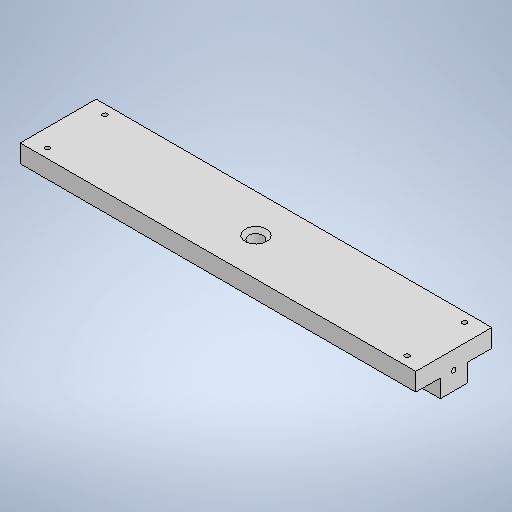
# Autodesk Inventor part: caster_holder
Saved by Autodesk Inventor 2026.3 (Build 303398000, 398)
## iProperties
Created: 2026-06-06
Part Number: caster_holder
Material: Generic
Document SubType Name: Modeling
Designer: gakut
Density: 1 g/cm^3
Appearance: Default
Author: gakut
## iProperties of the stored document caster_holder_3DPrint.ipt
Created: 2026-06-06
Part Number: caster_holder_3DPrint
Material: Generic
Document SubType Name: Modeling
Designer: gakut
Density: 1 g/cm^3
Appearance: Default
Author: gakut
Autodesk Inventor part; units mm, degrees
ref_plane "YZ Plane" through (0, 0, 0) normal (1, 0, 0) x (0, 1, 0)
ref_plane "XZ Plane" through (0, 0, 0) normal (0, 1, 0) x (-1, 0, 0)
ref_plane "XY Plane" through (0, 0, 0) normal (0, 0, 1) x (1, 0, 0)
sketch "Sketch1" plane through (0, 0, 0) normal (0, 1, 0) x (-1, 0, 0)
  line L0 (110, 21.125) -> (-110, 21.125)
  line L1 (-110, 21.125) -> (-110, -21.125)
  line L2 (-110, -21.125) -> (110, -21.125)
  line L3 (110, -21.125) -> (110, 21.125)
  line L4 (110, 21.125) -> (-110, -21.125) construction
  line L5 (-110, 21.125) -> (110, -21.125) construction
  point P0 (0, 0)
  dimension "d0" = 42.25
  dimension "d1" = 220
  constraints: 12 end point, 2 midpoint, 2 parallel, 1 horizontal, 1 perpendicular
  measures "d0" distance of L0.end L1.end
  measures "d1" distance of L0.start L0.end
extrude "Extrusion1" add sketch "Sketch1" along normal mid plane 20
sketch "Sketch2" plane through (0, 10, 0) normal (0, 1, 0) x (1, 0, 0)
  line L0 (110, 21.125) -> (-110, 21.125) projected
  line L1 (-110, -21.125) -> (110, -21.125) projected
  line L2 (-110, 21.125) -> (-110, -21.125) projected
  point P0 (0, 0)
  point P1 (-100, -16)
  point P2 (-100, 16)
  point P3 (-110, 0)
  dimension "d4" = 10
  dimension "d5" = 32
  dimension "d6" = 16
  constraints: 1 midpoint, 1 vertical alignment
  measures "d4" distance from line of L2 point (-100, 16)
  measures "d5" distance of point (-100, -16) point (-100, 16)
  measures "d6" vertical distance of point (-110, 0) point (-100, 16)
hole "Hole1" at (-100, 10, 16) at (-100, 10, -16) direction (0, -1, 0) diameter 2.6 end through all
mirror "Mirror1" about plane through (0, 0, 0) normal (1, 0, 0) of "Hole1"
sketch "Sketch4" plane through (0, 10, 0) normal (0, 1, 0) x (1, 0, 0)
  point P0 (0, 0)
  point P1 (0, 0)
  constraints: 1 coincident
hole "Hole2" at (0, 10, 0) direction (0, -1, 0) diameter 4.5 end through all counterbore diameter 8 counterbore depth 15
chamfer "Chamfer1" distance 2 angle 45 1 edges at (0, 10, -4)
sketch "Sketch6" plane through (110, -10, -21.125) normal (1, 0, 0) x (0, 0, -1)
  line L0 (-42.25, 20) -> (0, 20) projected
  line L1 (-28.625, 0) -> (-13.625, 0)
  line L2 (-13.625, 0) -> (-13.625, 20)
  line L3 (-13.625, 20) -> (-28.625, 20)
  line L4 (-28.625, 20) -> (-28.625, 0)
  line L5 (-28.625, 0) -> (-13.625, 20) construction
  line L6 (-13.625, 0) -> (-28.625, 20) construction
  line L7 (-42.25, 20) -> (-42.25, 0) projected
  line L8 (-42.25, 10) -> (0, 10)
  line L9 (0, 0) -> (0, 20) projected
  line L10 (0, 0) -> (0, 20) projected
  line L11 (-42.25, 20) -> (0, 20) projected
  line L12 (-42.25, 20) -> (-42.25, 0) projected
  line L13 (0, 0) -> (-42.25, 0) projected
  point P0 (-21.125, 10)
  point P1 (-13.625, 0)
  point P2 (-13.625, 10)
  point P3 (-28.625, 0)
  point P4 (-28.625, 10)
  dimension "d31" = 15
  constraints: 14 end point, 4 midpoint, 2 parallel, 1 horizontal, 1 perpendicular, 1 point on line
  measures "d31" distance between parallel lines of L4 L2
extrude "Extrusion4" cut sketch "Sketch6" against normal through all contours L8 L4 L13 L7 | L8 L9 L13 L2
sketch "Sketch7" plane through (110, 10, 21.125) normal (1, 0, 0) x (0, 0, -1)
  line L0 (0, -10) -> (13.625, -10) projected
  line L1 (28.625, -10) -> (42.25, -10) projected
  line L2 (0, 0) -> (0, -10) projected
  line L3 (42.25, -10) -> (42.25, 0) projected
  point P0 (21.125, -10)
  point P1 (6.8125, -5)
  point P2 (35.4375, -5)
  point P3 (6.8125, -10)
  point P4 (35.4375, -10)
  point P5 (0, -5)
  point P6 (42.25, -5)
  point P7 (21.125, -10)
  constraints: 4 midpoint, 2 horizontal alignment, 2 vertical alignment, 1 coincident
hole "Hole3" at (110, 0, 0) direction (-1, 0, 0) diameter 2.6 depth 5
mirror "Mirror2" about plane through (0, 0, 0) normal (1, 0, 0) of "Hole3"
equation "\"d6\" = 0.5 * d5"
body "Solid1"
